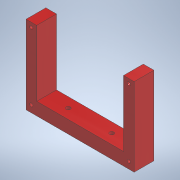
# Autodesk Inventor part: Vertical Electronics Spacer
Saved by Autodesk Inventor 2022 (Build 260153000, 153)
## iProperties
Created: 2021-11-02
Part Number: Vertical Electronics Spacer
Material: Generic
Document SubType Name: Modeling
Designer: Admin
Density: 1 g/cm^3
Appearance: Default
Author: Admin
Autodesk Inventor part; units mm, degrees
ref_plane "YZ Plane" through (0, 0, 0) normal (1, 0, 0) x (0, 1, 0)
ref_plane "XZ Plane" through (0, 0, 0) normal (0, 1, 0) x (-1, 0, 0)
ref_plane "XY Plane" through (0, 0, 0) normal (0, 0, 1) x (1, 0, 0)
sketch "Sketch1" plane through (0, 0, 0) normal (0, 0, 1) x (1, 0, 0)
  line L0 (0, 102.997) -> (0, 0)
  line L1 (0, 0) -> (142, 0)
  line L2 (142, 0) -> (142, 102.997)
  line L3 (142, 102.997) -> (128, 102.997)
  line L4 (128, 102.997) -> (128, 16.637)
  line L5 (128, 16.637) -> (14, 16.637)
  line L6 (14, 16.637) -> (14, 102.997)
  line L7 (14, 102.997) -> (0, 102.997)
  circle A0 centre (7, 96.997) radius 2.2
  circle A1 centre (135, 96.997) radius 2.2
  circle A2 centre (7, 8.997) radius 2.2
  circle A3 centre (135, 8.997) radius 2.2
  line L8 (14, 102.997) -> (128, 102.997)
  line L9 (28, 102.997) -> (114, 102.997)
  line L10 (114, 0) -> (28, 0)
  line L11 (135, 96.997) -> (135, 8.997) construction
  line L12 (7, 96.997) -> (7, 8.997) construction
  point P0 (71, 102.997)
  dimension "d0" = 102.997
  dimension "d3" = 14
  dimension "d4" = 86.36
  dimension "d44" = 4.4
  dimension "d45" = 4.4
  dimension "d46" = 128
  dimension "d47" = 7
  dimension "d48" = 14
  dimension "d49" = 7
  dimension "d50" = 114
  dimension "d51" = 4.4
  dimension "d52" = 4.4
  dimension "d53" = 88
  dimension "d54" = 88
  dimension "d55" = 6
  dimension "d56" = 6
  dimension "d84" = 128
  constraints: 26 end point, 6 perpendicular, 4 centre point, 3 parallel, 3 point on line, 2 midpoint, 2 vertical, 1 coincident, 1 collinear, 1 horizontal
  measures "d0" distance of L0.start L0.end
  measures "d3" distance of L6.end L0.start
  measures "d4" distance of L5.end L6.end
  measures "d44" diameter of A0
  measures "d45" diameter of A1
  measures "d46" distance of L12.start L11.start
  measures "d47" distance from line of L2 L11.start
  measures "d48" distance between parallel lines of L2 L4
  measures "d49" distance from line of L0 L12.start
  measures "d50" distance between parallel lines of L6 L4
  measures "d51" diameter of A2
  measures "d52" diameter of A3
  measures "d53" distance of L12.end L12.start
  measures "d54" distance of L11.end L11.start
  measures "d55" distance from line of L7 L12.start
  measures "d56" distance from line of L3 L11.start
  measures "d84" distance of L12.start L11.start
extrude "Extrusion1" add sketch "Sketch1" along normal blind 26 contours L7 L6 L5 L4 L3 L2 L1 L0
sketch "Sketch5" plane through (14, 16.637, 0) normal (0, 1, 0) x (1, 0, 0)
  line L0 (0, 0) -> (0, -26) projected
  line L1 (114, 0) -> (114, -26) projected
  line L2 (114, 0) -> (0, 0) construction
  line L3 (57, 0) -> (57, -26) construction
  line L4 (0, -13) -> (114, -13) construction
  circle A0 centre (28.425, -13) radius 2.75
  circle A1 centre (85.575, -13) radius 2.75
  point P0 (-14, 0)
  dimension "d57" = 5.5
  dimension "d58" = 28.575
  constraints: 4 end point, 3 midpoint, 2 centre point, 1 point on line, 1 symmetric about line, 1 vertical, 1 other
  measures "d57" diameter of A0
  measures "d58" distance from line of A0.centre L3
extrude "Extrusion2" cut sketch "Sketch5" against normal blind 26
equation "\"d3\" = d48"
equation "\"d44\" = d45"
equation "\"d47\" = 0.5 * d48"
equation "\"d49\" = 0.5 * d3"
equation "\"d51\" = d44"
equation "\"d52\" = d45"
equation "\"d54\" = d53"
equation "\"d56\" = d55"
body "Solid1"
